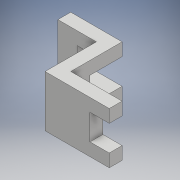
# Autodesk Inventor part: P3-6
Saved by Autodesk Inventor 2017 (Build 210142000, 142)
## iProperties
Created: 2017-02-12
Part Number: P3-6
Material: Generic
Document SubType Name: Modeling
Designer: Schaffel
Density: 1 g/cm^3
Appearance: Default
Author: Schaffel
Autodesk Inventor part; units mm, degrees
ref_plane "YZ Plane" through (0, 0, 0) normal (1, 0, 0) x (0, 1, 0)
ref_plane "XZ Plane" through (0, 0, 0) normal (0, 1, 0) x (-1, 0, 0)
ref_plane "XY Plane" through (0, 0, 0) normal (0, 0, 1) x (1, 0, 0)
sketch "Sketch1" plane through (0, 0, 0) normal (0, 1, 0) x (-1, 0, 0)
  line L0 (-40, 0) -> (-40, -40)
  line L1 (-40, -40) -> (-90, -40)
  line L2 (-90, -40) -> (-90, -30)
  line L3 (-90, -30) -> (-75, -30)
  line L4 (-75, -30) -> (-75, -10)
  line L5 (-75, -10) -> (-90, -10)
  line L6 (-90, -10) -> (-90, 0)
  line L7 (-90, 0) -> (-40, 0)
  point P0 (0, 0)
  constraints: 16 end point, 4 perpendicular, 2 point on line, 2 vertical, 1 parallel
extrude "Extrusion1" add sketch "Sketch1" along normal blind 10
sketch "Sketch2" plane through (0, 10, 0) normal (0, 1, 0) x (1, 0, 0)
  line L0 (40, 0) -> (40, 40) projected
  line L1 (40, 0) -> (40, 40)
  line L2 (40, 40) -> (50, 40)
  line L3 (40, 40) -> (90, 40) projected
  line L4 (50, 40) -> (50, 0)
  line L5 (50, 0) -> (40, 0)
  line L6 (40, 10) -> (50, 10)
  line L7 (40, 30) -> (50, 30)
  line L8 (40, 40) -> (40, 0) projected
  line L9 (40, 10) -> (40, 0)
  line L10 (40, 0) -> (50, 0)
  line L11 (50, 10) -> (50, 0)
  line L12 (40, 0) -> (90, 0) projected
  line L13 (50, 30) -> (50, 40)
  line L14 (90, 40) -> (40, 40) projected
  line L15 (40, 40) -> (50, 40)
  line L16 (40, 40) -> (40, 30)
  point P0 (0, 0)
  constraints: 24 end point, 5 collinear, 5 perpendicular, 5 point on line, 1 vertical
extrude "Extrusion2" add sketch "Sketch2" along normal blind 15
sketch "Sketch3" plane through (0, 25, 0) normal (0, 1, 0) x (1, 0, 0)
  line L0 (40, 0) -> (40, 40) projected
  line L1 (40, 0) -> (50, 0)
  line L2 (50, 0) -> (50, 10)
  line L3 (50, 10) -> (40, 10)
  line L4 (40, 10) -> (40, 0)
  line L5 (50, 40) -> (40, 40) projected
  line L6 (40, 40) -> (50, 40)
  line L7 (50, 40) -> (50, 30)
  line L8 (50, 40) -> (50, 0) projected
  line L9 (50, 30) -> (40, 30)
  line L10 (40, 30) -> (40, 40)
  point P0 (0, 0)
  constraints: 16 end point, 5 perpendicular, 3 point on line, 2 horizontal
extrude "Extrusion3" add sketch "Sketch3" along normal blind 25 contours L0 L3 L2 L1 | L0 L5 L7 L9
sketch "Sketch4" plane through (40, 0, -40) normal (-1, 0, 0) x (0, 0, 1)
  line L0 (0, 10) -> (0, 50) projected
  line L1 (10, 50) -> (0, 50) projected
  line L2 (0, 50) -> (10, 50)
  line L3 (10, 50) -> (10, 40)
  line L4 (10, 25) -> (10, 50) projected
  line L5 (10, 40) -> (0, 40)
  line L6 (0, 40) -> (0, 50)
  line L7 (40, 50) -> (30, 50) projected
  line L8 (30, 50) -> (40, 50)
  line L9 (40, 50) -> (40, 40)
  line L10 (40, 10) -> (40, 50) projected
  line L11 (40, 40) -> (30, 40)
  line L12 (30, 25) -> (30, 50) projected
  line L13 (30, 40) -> (30, 50)
  point P0 (40, 0)
  constraints: 16 end point, 6 point on line, 3 perpendicular, 1 collinear, 1 horizontal
extrude "Extrusion4" add sketch "Sketch4" along normal blind 15
sketch "Sketch5" plane through (25, 0, -40) normal (-1, 0, 0) x (0, 0, 1)
  line L0 (10, 50) -> (0, 50) projected
  line L1 (0, 50) -> (40, 50)
  line L2 (40, 50) -> (40, 40)
  line L3 (40, 40) -> (0, 40)
  line L4 (40, 40) -> (30, 40) projected
  line L5 (0, 50) -> (0, 40) projected
  line L6 (0, 40) -> (0, 50)
  point P0 (40, 0)
  constraints: 8 end point, 3 collinear, 1 perpendicular
extrude "Extrusion5" add sketch "Sketch5" along normal blind 15
body "Solid1"
